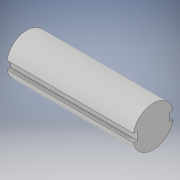
# Autodesk Inventor part: SpinnerAxelV1
Saved by Autodesk Inventor 2019 (Build 230136000, 136)
## iProperties
Created: 2018-07-30
Part Number: SpinnerAxelV1
Material: Generic
Document SubType Name: Modeling
Designer: Kitte_X
Density: 1 g/cm^3
Appearance: Default
Author: Kitte_X
Autodesk Inventor part; units mm, degrees
ref_plane "YZ Plane" through (0, 0, 0) normal (1, 0, 0) x (0, 1, 0)
ref_plane "XZ Plane" through (0, 0, 0) normal (0, 1, 0) x (-1, 0, 0)
ref_plane "XY Plane" through (0, 0, 0) normal (0, 0, 1) x (1, 0, 0)
sketch "Sketch1" plane through (0, 0, 0) normal (1, 0, 0) x (0, 1, 0)
  line L0 (5, 20) -> (-5, 20)
  line L1 (5, -20) -> (-5, -20)
  arc A0 (5, -24.4949) -> (5, 24.4949) centre (0, 0) ccw
  arc A1 (-5, 24.4949) -> (-5, -24.4949) centre (0, 0) ccw
  line L2 (5, 24.4949) -> (5, 20)
  line L3 (5, -20) -> (5, -24.4949)
  line L4 (-5, -24.4949) -> (-5, -20)
  line L5 (-5, 20) -> (-5, 24.4949)
  dimension "d3" = 20
  dimension "d4" = 40
  dimension "d7" = 25
  dimension "d8" = 25
  dimension "d9" = 10
  constraints: 12 end point, 4 parallel, 4 perpendicular, 4 point on circle, 2 centre point, 2 vertical, 1 coincident
  measures "d3" distance from line of L0 point (0, 0)
  measures "d4" distance between parallel lines of L0 L1
  measures "d7" radius of A0
  measures "d8" radius of A1
  measures "d9" distance between parallel lines of L5 L2
extrude "Extrusion1" add sketch "Sketch1" along normal blind 156
body "Solid1"
